Autodesk Fusion 360 part; units mm, degrees
note: some values were not read from the file. Chosen so that the rebuilt part matches the saved one: which bodies a step acts on.
(part 2 of 2)
sketch "Sketch603" plane through (0, 0, 0) normal (0, 0, 1) x (1, 0, 0)
  line L0 (12.35, 93.33) -> (14.95, 93.33)
  line L1 (14.95, 93.33) -> (14.95, 95.95)
  line L2 (14.95, 95.95) -> (12.35, 95.95)
  line L3 (12.35, 95.95) -> (12.35, 93.33)
  line L4 (69.5, 93.33) -> (72.1, 93.33)
  line L5 (72.1, 93.33) -> (72.1, 95.95)
  line L6 (72.1, 95.95) -> (69.5, 95.95)
  line L7 (69.5, 95.95) -> (69.5, 93.33)
extrude "Extrude597" cut sketch "Sketch603" along normal blind 3 from surface at -0.5 bodies 85
move_body "Move652" bodies 85 to x (1, 0, 0) y (0, 0.994522, 0.104528) z (0, -0.104528, 0.994522) at (0, 0, 14.5)
named bodies: "Bottom Plate", "Top Plate"
